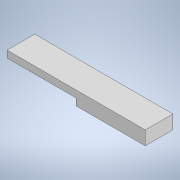
# Autodesk Inventor part: 3D_Domain
Saved by Autodesk Inventor 2021 (Build 250183000, 183)
## iProperties
Created: 2022-12-14
Part Number: 3D_Domain
Material: Genérico
Document SubType Name: Modeling
Designer: achom
Density: 1 g/cm^3
Appearance: Valor por defecto
Author: achom
Autodesk Inventor part; units mm, degrees
ref_plane "YZ Plane" through (0, 0, 0) normal (1, 0, 0) x (0, 1, 0)
ref_plane "XZ Plane" through (0, 0, 0) normal (0, 1, 0) x (-1, 0, 0)
ref_plane "XY Plane" through (0, 0, 0) normal (0, 0, 1) x (1, 0, 0)
sketch "Boceto2" plane through (0, 0, 0) normal (0, 0, 1) x (1, 0, 0)
  line L0 (0, 0) -> (2000, 0)
  line L1 (2000, 0) -> (2000, 200)
  line L2 (2000, 200) -> (0, 200)
  line L3 (0, 200) -> (0, 0)
  line L4 (0, 0) -> (1000, 0)
  line L5 (1000, 0) -> (1000, 100)
  line L6 (1000, 100) -> (0, 100)
  line L7 (0, 100) -> (0, 0)
  dimension "d0" = 2000
  dimension "d1" = 200
  dimension "d2" = 1000
  dimension "d3" = 100
  constraints: 16 end point, 4 parallel, 2 horizontal, 2 perpendicular
  measures "d0" distance of L2.end L1.end
  measures "d1" distance of L1.end L0.end
  measures "d2" distance of L6.end L5.end
  measures "d3" distance of L5.end L4.end
extrude "Extrusión1" add sketch "Boceto2" along normal blind 400 contours L5 L6 L3 L2 L1 L0
